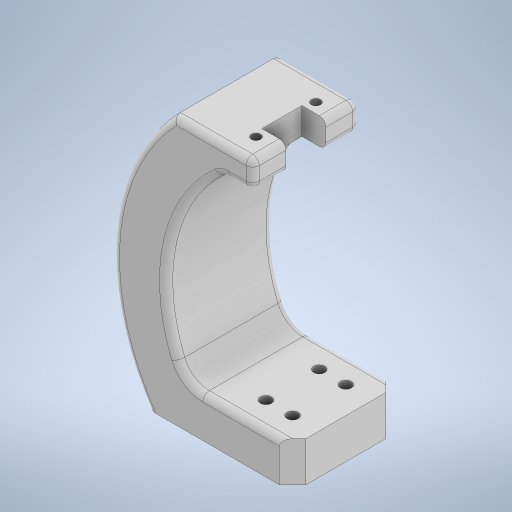
# Autodesk Inventor part: Gestell
Saved by Autodesk Inventor 2024 (Build 280153000, 153)
## iProperties
Created: 2023-05-12
Part Number: Gestell
Material: Generic
Document SubType Name: Modeling
Designer: Raj
Density: 1 g/cm^3
Appearance: Default
Author: Raj
Autodesk Inventor part; units mm, degrees
note: some values were not read from the file. Chosen so that the rebuilt part matches the saved one: direction of "Hole1".
ref_plane "YZ Plane" through (0, 0, 0) normal (1, 0, 0) x (0, 1, 0)
ref_plane "XZ Plane" through (0, 0, 0) normal (0, 1, 0) x (-1, 0, 0)
ref_plane "XY Plane" through (0, 0, 0) normal (0, 0, 1) x (1, 0, 0)
sketch "Sketch1" plane through (0, 0, 0) normal (0, 1, 0) x (-1, 0, 0)
  line L0 (0, 0) -> (0, 30)
  line L1 (0, 30) -> (67.4986, 30)
  line L2 (0, 0) -> (108.6263, 0)
  arc A0 (85.9984, 42.4) -> (54.9868, 177.4545) centre (-25, 88) ccw
  arc A1 (108.6263, 0) -> (89.2629, 200) centre (-25, 88) ccw
  line L3 (30, 200) -> (89.2629, 200)
  line L4 (30, 180) -> (48.3212, 180)
  line L5 (30, 200) -> (30, 180)
  arc A2 (67.4986, 30) -> (85.9984, 42.4) centre (67.4986, 50) ccw
  arc A3 (54.9868, 177.4545) -> (48.3212, 180) centre (48.3212, 170) ccw
  point P0 (52.0454, 180)
  point P1 (80.0524, 30)
  dimension "d0" = 30
  dimension "d1" = 240
  dimension "d2" = 320
  dimension "d3" = 25
  dimension "d4" = 88
  dimension "d5" = 200
  dimension "d6" = 180
  dimension "d7" = 30
  dimension "d8" = 20
  dimension "d9" = 10
  constraints: 12 end point, 10 point on circle, 4 centre point, 4 tangent, 3 horizontal, 2 point on line, 2 vertical, 1 coincident, 1 perpendicular
  measures "d0" distance of L0.start L0.end
  measures "d1" diameter of A0
  measures "d2" diameter of A1
  measures "d3" horizontal distance of L0.start A0.centre
  measures "d4" vertical distance of L0.start A0.centre
  measures "d5" distance from line of L0.start L3
  measures "d6" distance from line of L0.start L4
  measures "d7" distance from line of L0.start L5
  measures "d8" radius of A2
  measures "d9" radius of A3
extrude "Extrusion1" add sketch "Sketch1" along normal mid plane 80
sketch "Sketch2" plane through (0, 40, 0) normal (0, 0, -1) x (-1, 0, 0)
  line L0 (0, -80) -> (0, 0) projected
  line L1 (0, 0) -> (108.6263, 0) projected
  point P0 (0, -40)
  point P1 (20, -20)
  point P2 (40, -20)
  point P3 (20, -60)
  point P4 (40, -60)
  dimension "d12" = 20
  dimension "d13" = 20
  dimension "d16" = 20
  dimension "d19" = 40
  constraints: 1 horizontal, 1 vertical, 3 other
  measures "d12" distance from line of point (20, -20) L0
  measures "d13" distance from line of point (20, -20) L1
  measures "d16" distance of point (20, -20) point (40, -20)
  measures "d19" distance of point (20, -20) point (20, -60)
hole "Hole1" at (-20, 20, 0) at (-40, 20, 0) at (-20, -20, 0) at (-40, -20, 0) direction (0, 0, 1) diameter 8.4 depth 30 counterbore diameter 15 counterbore depth 8
sketch "Sketch3" plane through (-89.2629, 40, 200) normal (0, 0, 1) x (1, 0, 0)
  line L0 (89.2629, -80) -> (89.2629, 0) projected
  line L1 (0, 0) -> (59.2629, 0) projected
  point P0 (89.2629, -40)
  point P1 (44.2629, -17.5)
  point P2 (44.2629, -62.5)
  dimension "d29" = 45
  dimension "d30" = 45
  dimension "d31" = 45
  dimension "d32" = 17.5
  measures "d29" distance from line of L0 point (44.263, -17.5)
  measures "d30" distance from line of L0 point (44.263, -62.5)
  measures "d31" distance of point (44.263, -62.5) point (44.263, -17.5)
  measures "d32" distance from line of L1 point (44.263, -17.5)
hole "Hole2" at (-45, 22.5, 200) at (-45, -22.5, 200) direction (0, 0, -1) diameter 6.917 depth 12 tip angle 118 thread size "M8x1" class "6H" standard "ISO Metric profile"
sketch "Sketch4" plane through (-89.2629, 40, 200) normal (0, 0, 1) x (1, 0, 0)
  line L0 (41.2629, -55) -> (59.2629, -55)
  line L1 (59.2629, -55) -> (59.2629, -25)
  line L2 (59.2629, -25) -> (41.2629, -25)
  line L3 (41.2629, -25) -> (41.2629, -55)
  line L4 (41.2629, -55) -> (59.2629, -25) construction
  line L5 (59.2629, -55) -> (41.2629, -25) construction
  line L6 (59.2629, -80) -> (59.2629, 0) projected
  line L7 (0, 0) -> (59.2629, 0) projected
  point P0 (89.2629, -40)
  point P1 (50.2629, -40)
  dimension "d40" = 18
  dimension "d41" = 30
  dimension "d42" = 0
  dimension "d43" = 40
  constraints: 12 end point, 2 midpoint, 2 parallel, 1 horizontal, 1 perpendicular
  measures "d40" distance of L2.end L1.end
  measures "d41" distance of L1.end L0.end
  measures "d42" distance between parallel lines of L1 L6
  measures "d43" distance from line of L7 point (50.263, -40)
extrude "Extrusion2" cut sketch "Sketch4" against normal up to surface (20 mm away)
chamfer "Chamfer1" distance 10 angle 45 2 edges at (0, -40, 15) (0, 40, 15)
fillet "Fillet1" radius 5 20 edges at (-30, -27.5, 200) (-30, -40, 190) (-78.6342, -40, 33.3868) (-91.9563, -40, 114.8558) (-51.8887, -40, 179.342) (-39.1606, -40, 180) (-38.7493, -40, 30) (-30, 27.5, 200) (-30, 40, 190) (-30, -27.5, 180) (-30, 27.5, 180) (-78.6342, 40, 33.3868) (-91.9563, 40, 114.8558) (-51.8887, 40, 179.342) (-39.1606, 40, 180) (-38.7493, 40, 30) (-59.6314, 40, 200) (-59.6314, -40, 200) (-134.2553, 40, 103.4187) (-134.2553, -40, 103.4187)
body "Solid1"
